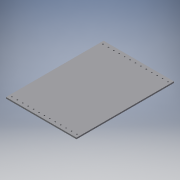
# Autodesk Inventor part: KrackenPlate1
Saved by Autodesk Inventor 2016 (Build 200138000, 138)
## iProperties
Created: 2015-09-01
Part Number: KrackenPlate1
Material: Generic
Document SubType Name: Modeling
Designer: Tim
Density: 1 g/cm^3
Appearance: Default
Author: Tim
Autodesk Inventor part; units mm, degrees
ref_plane "YZ Plane" through (0, 0, 0) normal (1, 0, 0) x (0, 1, 0)
ref_plane "XZ Plane" through (0, 0, 0) normal (0, 1, 0) x (-1, 0, 0)
ref_plane "XY Plane" through (0, 0, 0) normal (0, 0, 1) x (1, 0, 0)
sketch "Sketch1" plane through (0, 0, 0) normal (0, 1, 0) x (-1, 0, 0)
  line L0 (104, -144) -> (-104, -144)
  line L1 (-104, -144) -> (-104, 144)
  line L2 (-104, 144) -> (104, 144)
  line L3 (104, 144) -> (104, -144)
  line L4 (104, -144) -> (-104, 144) construction
  line L5 (-104, -144) -> (104, 144) construction
  circle A0 centre (96, 134.4) radius 1.85 projected
  circle A1 centre (80, 134.4) radius 1.85 projected
  circle A2 centre (64, 134.4) radius 1.85 projected
  circle A3 centre (48, 134.4) radius 1.85 projected
  circle A4 centre (32, 134.4) radius 1.85 projected
  circle A5 centre (16, 134.4) radius 1.85 projected
  circle A6 centre (0, 134.4) radius 1.85 projected
  circle A7 centre (-16, 134.4) radius 1.85 projected
  circle A8 centre (-32, 134.4) radius 1.85 projected
  circle A9 centre (-48, 134.4) radius 1.85 projected
  circle A10 centre (-64, 134.4) radius 1.85 projected
  circle A11 centre (-80, 134.4) radius 1.85 projected
  circle A12 centre (-96, 134.4) radius 1.85 projected
  line L6 (104, 144) -> (-104, -144) construction
  line L7 (-104, 144) -> (104, -144) construction
  circle A13 centre (96, -134.4) radius 1.85
  circle A14 centre (80, -134.4) radius 1.85
  circle A15 centre (64, -134.4) radius 1.85
  circle A16 centre (48, -134.4) radius 1.85
  circle A17 centre (32, -134.4) radius 1.85
  circle A18 centre (16, -134.4) radius 1.85
  circle A19 centre (0, -134.4) radius 1.85
  circle A20 centre (-16, -134.4) radius 1.85
  circle A21 centre (-32, -134.4) radius 1.85
  circle A22 centre (-48, -134.4) radius 1.85
  circle A23 centre (-64, -134.4) radius 1.85
  circle A24 centre (-80, -134.4) radius 1.85
  circle A25 centre (-96, -134.4) radius 1.85
  point P0 (0, 0)
  dimension "d0" = 208
  dimension "d1" = 288
  constraints: 16 end point, 2 midpoint, 2 parallel, 1 horizontal, 1 perpendicular
  measures "d0" distance of L1.end L2.end
  measures "d1" distance of L2.end L0.start
extrude "Extrusion4" add sketch "Sketch1" along normal blind 4
body "Solid4"
